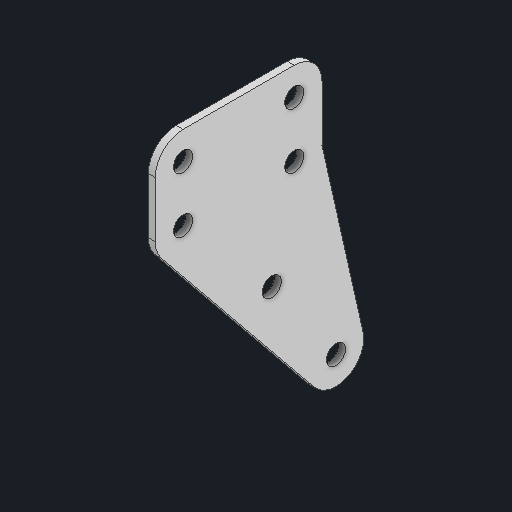
# Autodesk Inventor part: Angle Brace Gusset
Saved by Autodesk Inventor 2025 (Build 290162000, 162)
## iProperties
Created: 2024-10-13
Part Number: Angle Brace Gusset
Material: Generic
Document SubType Name: Modeling
Designer: Averey Ku
Density: 1 g/cm^3
Appearance: Default
d0: 0.500 in
d6: 0.172 in
d9: 0.500 in
d10: 1.000 in
d11: 0.500 in
d12: 1.000 in
Author: Averey Ku
Autodesk Inventor part; units mm, degrees
ref_plane "YZ Plane" through (0, 0, 0) normal (1, 0, 0) x (0, 1, 0)
ref_plane "XZ Plane" through (0, 0, 0) normal (0, 1, 0) x (-1, 0, 0)
ref_plane "XY Plane" through (0, 0, 0) normal (0, 0, 1) x (1, 0, 0)
sketch "maiin" plane through (0, 0, 0) normal (0, 0, 1) x (1, 0, 0)
  circle A0 centre (-6.5018, 3.4753) radius 2.1844
  line L0 (-31.2537, -6.2516) -> (11.7059, 28.671)
  circle A1 centre (-27.2482, -11.1789) radius 2.1844
  arc A2 (-31.2537, -6.2516) -> (-25.8521, -17.3735) centre (-27.2482, -11.1789) ccw
  line L1 (34.75, -1.6563) -> (34.75, 23.7437)
  line L2 (15.7114, 30.0937) -> (28.4, 30.0937)
  circle A3 centre (28.4114, 23.7437) radius 2.1844
  circle A4 centre (28.4, -1.6563) radius 2.1844
  circle A5 centre (15.7114, 23.7437) radius 2.1844
  circle A6 centre (15.7, -1.6563) radius 2.1844
  arc A7 (34.75, 23.7437) -> (28.4, 30.0937) centre (28.4, 23.7437) ccw
  arc A8 (15.7114, 30.0937) -> (11.7059, 28.671) centre (15.7114, 23.7437) ccw
  arc A9 (28.4, -8.0063) -> (34.75, -1.6563) centre (28.4, -1.6563) ccw
  line L3 (28.4, -8.0063) -> (15.7114, -8.0063)
  line L4 (15.7114, -8.0063) -> (-25.8521, -17.3735)
  point P0 (10.0881, 4.3711)
  point P1 (32.8902, 28.2338)
  dimension "d0" = 12.7
  dimension "d6" = 4.3688
  dimension "d9" = 12.7
  dimension "d10" = 25.4
  dimension "d11" = 12.7
  dimension "d12" = 25.4
  measures "d0" diameter of A2
  measures "d6" diameter of A6
  measures "d9" distance of A4.centre A6.centre
  measures "d10" distance of A4.centre A7.centre
  measures "d11" distance of A8.centre A3.centre
  measures "d12" distance of A6.centre A8.centre
sketch "Sketch1" plane through (0, 0, 0) normal (1, 0, 0) x (0, 1, 0)
  circle A0 centre (-34.9132, -20.2684) radius 2.1844
  line L0 (-59.6651, -29.9953) -> (-16.7055, 4.9273)
  circle A1 centre (-55.6596, -34.9226) radius 2.1844
  arc A2 (-59.6651, -29.9953) -> (-54.2635, -41.1172) centre (-55.6596, -34.9226) ccw
  line L1 (6.3386, -25.4) -> (6.3386, 0)
  line L2 (-12.7, 6.35) -> (-0.0114, 6.35)
  circle A3 centre (0, 0) radius 2.1844
  circle A4 centre (-0.0114, -25.4) radius 2.1844
  circle A5 centre (-12.7, 0) radius 2.1844
  circle A6 centre (-12.7114, -25.4) radius 2.1844
  arc A7 (6.3386, 0) -> (-0.0114, 6.35) centre (-0.0114, 0) ccw
  arc A8 (-12.7, 6.35) -> (-16.7055, 4.9273) centre (-12.7, 0) ccw
  arc A9 (-0.0114, -31.75) -> (6.3386, -25.4) centre (-0.0114, -25.4) ccw
  line L3 (-0.0114, -31.75) -> (-12.7, -31.75)
  line L4 (-12.7, -31.75) -> (-54.2635, -41.1172)
  constraints: 1 other
extrude "Extrusion1" add sketch "Sketch1" along normal blind 1.5875
body "Solid1"
